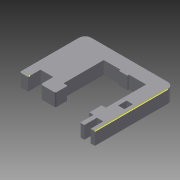
# Autodesk Inventor part: Gripper V 8.0 servo bracket side 6mm
Saved by Autodesk Inventor 2015 (Build 190159000, 159)
## iProperties
Created: 2015-06-23
Part Number: Gripper V 8.0 servo bracket side 6mm
Material: Generic
Document SubType Name: Modeling
Designer: Stackpole
Density: 1 g/cm^3
Appearance: Default
Author: Stackpole
Autodesk Inventor part; units mm, degrees
ref_plane "YZ Plane" through (0, 0, 0) normal (1, 0, 0) x (0, 1, 0)
ref_plane "XZ Plane" through (0, 0, 0) normal (0, 1, 0) x (-1, 0, 0)
ref_plane "XY Plane" through (0, 0, 0) normal (0, 0, 1) x (1, 0, 0)
sketch "Sketch1" plane through (0, 0, 0) normal (0, 0, 1) x (1, 0, 0)
  line L0 (0.081, -0.7334) -> (0.081, 5.1966)
  line L1 (0.081, 5.1966) -> (6.081, 5.1966)
  line L2 (6.081, 5.1966) -> (6.081, -0.7334)
  line L3 (38.07, 30.2666) -> (-3.919, 30.2666)
  line L4 (-3.919, 30.2666) -> (-3.919, -0.7334)
  line L5 (-3.919, -0.7334) -> (0.081, -0.7334)
  line L6 (31.07, 24.0666) -> (23.025, 24.0666)
  line L7 (23.025, 24.0666) -> (23.025, 23.2666)
  line L8 (23.025, 23.2666) -> (19.0255, 23.2666)
  line L9 (19.0255, 23.2666) -> (19.0255, 24.0666)
  line L10 (19.0255, 24.0666) -> (11.081, 24.0666)
  line L11 (38.07, 30.2666) -> (38.07, -7.113)
  line L12 (11.081, 24.0666) -> (11.081, 5.07)
  line L13 (11.081, 5.07) -> (13.0755, 5.07)
  line L14 (13.0755, 5.07) -> (13.0755, -0.7334)
  line L15 (6.081, -0.7334) -> (13.0755, -0.7334)
  line L16 (31.07, 24.0666) -> (31.07, 5.07)
  line L17 (31.07, 5.07) -> (29.0755, 5.07)
  line L18 (29.0755, 5.07) -> (29.0755, -0.7334)
  line L19 (29.0755, -0.7334) -> (31.07, -0.7334)
  line L20 (31.07, -0.7334) -> (31.07, -7.113)
  line L21 (38.07, -7.113) -> (31.07, -7.113)
  dimension "d0" = 6
  dimension "d2" = 31
  dimension "d4" = 19.989
  dimension "d10" = 4
  dimension "d13" = 3.9995
  dimension "d15" = 0.8
  dimension "d21" = 6.2
  dimension "d22" = 25.07
  dimension "d38" = 31
  dimension "d41" = 5
  dimension "d43" = 1.9945
  dimension "d45" = 5.8034
  dimension "d46" = 37.3796
  dimension "d47" = 7
  constraints: 44 end point, 12 perpendicular, 5 vertical, 4 horizontal, 3 collinear, 1 point on line
  measures "d0" distance of L0.end L1.end
  measures "d2" distance of L3.end L4.end
  measures "d4" distance of L10.end L6.start
  measures "d10" distance of L4.end L0.start
  measures "d13" distance of L7.end L8.end
  measures "d15" distance of L8.end L9.end
  measures "d21" distance between parallel lines of L3 L10
  measures "d22" distance between parallel lines of L3 L1
  measures "d38" distance between parallel lines of L3 L15
  measures "d41" distance between parallel lines of L2 L12
  measures "d43" distance of L16.end L17.end
  measures "d45" distance of L13.end L14.end
  measures "d46" distance between parallel lines of L3 L21
  measures "d47" distance between parallel lines of L11 L16
extrude "Extrusion1" add sketch "Sketch1" along normal blind 6
fillet "Fillet1" radius 3 2 edges at (-3.919, 30.2666, 3) (38.07, 30.2666, 3)
fillet "Fillet2" radius 0.9 2 edges at (-3.919, -0.7334, 3) (6.081, -0.7334, 3)
sketch "Sketch2" plane through (0, 0, 6) normal (0, 0, 1) x (1, 0, 0)
  line L0 (38.07, -7.113) -> (38.07, 27.2666) projected
  point P0 (0, 0)
sketch "Sketch3" plane through (0, 0, 0) normal (0, 0, -1) x (-1, 0, 0)
  line L0 (-33.07, -7.113) -> (-36.07, -7.113)
  line L1 (-36.07, -7.113) -> (-36.07, -1.113)
  line L2 (-36.07, -1.113) -> (-33.07, -1.113)
  line L3 (-33.07, -1.113) -> (-33.07, -7.113)
  line L4 (-33.07, -13.494) -> (-36.07, -13.494) projected
  line L5 (-38.07, -7.113) -> (-38.07, 27.2666) projected
  line L6 (-35.07, 30.2666) -> (0.919, 30.2666) projected
  line L7 (-31.07, -7.113) -> (-38.07, -7.113) projected
  point P0 (0, 0)
  dimension "d31" = 3
  dimension "d32" = 6
  dimension "d34" = 2
  constraints: 8 end point, 2 parallel, 1 collinear, 1 horizontal, 1 perpendicular
  measures "d31" distance of L1.end L2.end
  measures "d32" distance of L2.end L0.start
  measures "d34" distance between parallel lines of L5 L1
extrude "Extrusion2" cut sketch "Sketch3" against normal blind 10
fillet "Fillet4" radius 0.5 4 edges at (13.0755, -0.7334, 3) (31.07, -7.113, 3) (13.0755, 5.07, 3) (29.0755, 5.07, 3)
sketch "Sketch4" plane through (0, 0, 6) normal (0, 0, 1) x (1, 0, 0)
  line L0 (33.07, 12.887) -> (36.07, 12.887)
  line L1 (36.07, 12.887) -> (36.07, 8.887)
  line L2 (36.07, 8.887) -> (33.07, 8.887)
  line L3 (33.07, 8.887) -> (33.07, 12.887)
  line L4 (31.07, 24.0666) -> (31.07, 5.07) projected
  line L5 (33.07, -1.113) -> (36.07, -1.113) projected
  point P0 (0, 0)
  dimension "d48" = 3
  dimension "d49" = 2
  dimension "d50" = 4
  dimension "d53" = 10
  constraints: 8 end point, 2 parallel, 1 horizontal, 1 perpendicular
  measures "d48" distance of L0.start L0.end
  measures "d49" distance between parallel lines of L4 L3
  measures "d50" distance of L0.end L1.end
  measures "d53" distance between parallel lines of L2 L5
extrude "Extrusion3" cut sketch "Sketch4" against normal blind 10
body "Solid1"
